Autodesk Fusion 360 part; units mm, degrees
(part 2 of 2)
  line L885 (21.4286, -124.7042) -> (15.7857, -127.9621)
  line L886 (15.7857, -127.9621) -> (15.7857, -134.4779)
  line L887 (21.4286, -137.7358) -> (27.0714, -134.4779)
  line L888 (15.7857, -134.4779) -> (21.4286, -137.7358)
  line L889 (8.6429, -140.3339) -> (8.6429, -146.5)
  line L890 (19.9286, -146.5) -> (19.9286, -140.3339)
  line L891 (14.2857, -137.076) -> (8.6429, -140.3339)
  line L892 (19.9286, -140.3339) -> (14.2857, -137.076)
  line L893 (41.3571, -134.4779) -> (41.3571, -127.9621)
  line L894 (41.3571, -127.9621) -> (35.7143, -124.7042)
  line L895 (35.7143, -124.7042) -> (30.0714, -127.9621)
  line L896 (30.0714, -127.9621) -> (30.0714, -134.4779)
  line L897 (35.7143, -137.7358) -> (41.3571, -134.4779)
  line L898 (30.0714, -134.4779) -> (35.7143, -137.7358)
  line L899 (22.9286, -140.3339) -> (22.9286, -146.5)
  line L900 (34.2143, -146.5) -> (34.2143, -140.3339)
  line L901 (28.5714, -137.076) -> (22.9286, -140.3339)
  line L902 (34.2143, -140.3339) -> (28.5714, -137.076)
  line L903 (55.6428, -134.4779) -> (55.6428, -127.9621)
  line L904 (55.6428, -127.9621) -> (50, -124.7042)
  line L905 (50, -124.7042) -> (44.3571, -127.9621)
  line L906 (44.3571, -127.9621) -> (44.3571, -134.4779)
  line L907 (50, -137.7358) -> (55.6428, -134.4779)
  line L908 (44.3571, -134.4779) -> (50, -137.7358)
  line L909 (37.2143, -140.3339) -> (37.2143, -146.5)
  line L910 (45.9892, -148.2993) -> (48.5, -146.8497)
  line L911 (48.5, -146.8497) -> (48.5, -140.3339)
  line L912 (42.8571, -137.076) -> (37.2143, -140.3339)
  line L913 (48.5, -140.3339) -> (42.8571, -137.076)
  line L914 (69.9286, -134.4779) -> (69.9286, -127.9621)
  line L915 (69.9286, -127.9621) -> (64.2857, -124.7042)
  line L916 (64.2857, -124.7042) -> (58.6429, -127.9621)
  line L917 (58.6429, -127.9621) -> (58.6429, -134.4779)
  line L918 (64.2857, -137.7358) -> (69.9286, -134.4779)
  line L919 (58.6429, -134.4779) -> (64.2857, -137.7358)
  line L920 (51.5, -140.3339) -> (51.5, -146.8497)
  line L921 (51.5, -146.8497) -> (57.1429, -150.1076)
  line L922 (57.1429, -150.1076) -> (62.7857, -146.8497)
  line L923 (62.7857, -146.8497) -> (62.7857, -140.3339)
  line L924 (57.1429, -137.076) -> (51.5, -140.3339)
  line L925 (62.7857, -140.3339) -> (57.1429, -137.076)
  line L926 (84.2142, -134.4779) -> (84.2142, -127.9621)
  line L927 (78.5715, -124.7041) -> (72.9286, -127.9621)
  line L928 (72.9286, -127.9621) -> (72.9286, -134.4779)
  line L929 (78.5714, -137.7358) -> (84.2142, -134.4779)
  line L930 (72.9286, -134.4779) -> (78.5714, -137.7358)
  line L931 (65.7857, -140.3339) -> (65.7857, -146.8497)
  line L932 (65.7857, -146.8497) -> (71.4286, -150.1076)
  line L933 (71.4286, -150.1076) -> (77.0714, -146.8497)
  line L934 (77.0714, -146.8497) -> (77.0714, -140.3339)
  line L935 (71.4286, -137.076) -> (65.7857, -140.3339)
  line L936 (77.0714, -140.3339) -> (71.4286, -137.076)
  line L937 (98.5, -134.4779) -> (98.5, -127.9621)
  line L938 (98.5, -127.9621) -> (92.8572, -124.7042)
  line L939 (87.2142, -127.9621) -> (87.2142, -134.4779)
  line L940 (92.8571, -137.7358) -> (98.5, -134.4779)
  line L941 (87.2142, -134.4779) -> (92.8571, -137.7358)
  line L942 (80.0714, -140.3339) -> (80.0714, -146.8497)
  line L943 (80.0714, -146.8497) -> (85.7143, -150.1076)
  line L944 (85.7143, -150.1076) -> (91.3571, -146.8497)
  line L945 (91.3571, -146.8497) -> (91.3571, -140.3339)
  line L946 (85.7143, -137.076) -> (80.0714, -140.3339)
  line L947 (91.3571, -140.3339) -> (85.7143, -137.076)
  line L948 (94.3571, -140.3339) -> (94.3571, -146.8497)
  line L949 (94.3571, -146.8497) -> (100, -150.1076)
  line L950 (100, -137.076) -> (94.3571, -140.3339)
  line L951 (-87.2143, -154.113) -> (-87.2143, -152.7061)
  line L952 (-87.2143, -152.7061) -> (-92.8572, -149.4482)
  line L953 (-92.8572, -149.4482) -> (-98.143, -152.5)
  line L954 (-72.9286, -159.2219) -> (-72.9286, -152.7061)
  line L955 (-72.9286, -152.7061) -> (-78.5714, -149.4482)
  line L956 (-78.5714, -149.4482) -> (-84.2143, -152.7061)
  line L957 (-84.2143, -152.7061) -> (-84.2143, -159.2219)
  line L958 (-78.5714, -162.4798) -> (-72.9286, -159.2219)
  line L959 (-84.2143, -159.2219) -> (-78.5714, -162.4798)
  line L960 (-80.0714, -170.5) -> (-80.0714, -165.0779)
  line L961 (-80.0714, -165.0779) -> (-85, -162.2324)
  line L962 (-58.6429, -159.2219) -> (-58.6429, -152.7061)
  line L963 (-58.6429, -152.7061) -> (-64.2857, -149.4482)
  line L964 (-64.2857, -149.4482) -> (-69.9286, -152.7061)
  line L965 (-69.9286, -152.7061) -> (-69.9286, -159.2219)
  line L966 (-64.2857, -162.4798) -> (-58.6429, -159.2219)
  line L967 (-69.9286, -159.2219) -> (-64.2857, -162.4798)
  line L968 (-77.0714, -165.0779) -> (-77.0714, -170.5)
  line L969 (-65.7857, -170.5) -> (-65.7857, -165.0779)
  line L970 (-71.4286, -161.82) -> (-77.0714, -165.0779)
  line L971 (-65.7857, -165.0779) -> (-71.4286, -161.82)
  line L972 (-47.6236, -150.8202) -> (-50, -149.4482)
  line L973 (-50, -149.4482) -> (-55.6429, -152.7061)
  line L974 (-55.6429, -152.7061) -> (-55.6429, -159.2219)
  line L975 (-50, -162.4798) -> (-48, -161.3251)
  line L976 (-55.6429, -159.2219) -> (-50, -162.4798)
  line L977 (-62.7857, -165.0779) -> (-62.7857, -170.5)
  line L978 (-51.5, -170.5) -> (-51.5, -165.0779)
  line L979 (-57.1429, -161.82) -> (-62.7857, -165.0779)
  line L980 (-51.5, -165.0779) -> (-57.1429, -161.82)
  line L981 (-48.5, -165.0779) -> (-48.5, -170.5)
  line L982 (55.6428, -159.2219) -> (55.6428, -152.7061)
  line L983 (55.6428, -152.7061) -> (50, -149.4482)
  line L984 (50, -149.4482) -> (47.6236, -150.8202)
  line L985 (50, -162.4798) -> (55.6428, -159.2219)
  line L986 (48, -161.3251) -> (50, -162.4798)
  line L987 (48.5, -170.5) -> (48.5, -165.0779)
  line L988 (69.9286, -159.2219) -> (69.9286, -152.7061)
  line L989 (69.9286, -152.7061) -> (64.2857, -149.4482)
  line L990 (64.2857, -149.4482) -> (58.6429, -152.7061)
  line L991 (58.6429, -152.7061) -> (58.6429, -159.2219)
  line L992 (64.2857, -162.4798) -> (69.9286, -159.2219)
  line L993 (58.6429, -159.2219) -> (64.2857, -162.4798)
  line L994 (51.5, -165.0779) -> (51.5, -170.5)
  line L995 (62.7857, -170.5) -> (62.7857, -165.0779)
  line L996 (57.1429, -161.82) -> (51.5, -165.0779)
  line L997 (62.7857, -165.0779) -> (57.1429, -161.82)
  line L998 (84.2143, -159.2219) -> (84.2143, -152.7061)
  line L999 (84.2143, -152.7061) -> (78.5714, -149.4482)
  line L1000 (78.5714, -149.4482) -> (72.9286, -152.7061)
  line L1001 (72.9286, -152.7061) -> (72.9286, -159.2219)
  line L1002 (78.5714, -162.4798) -> (84.2143, -159.2219)
  line L1003 (72.9286, -159.2219) -> (78.5714, -162.4798)
  line L1004 (65.7857, -165.0779) -> (65.7857, -170.5)
  line L1005 (77.0714, -170.5) -> (77.0714, -165.0779)
  line L1006 (71.4286, -161.82) -> (65.7857, -165.0779)
  line L1007 (77.0714, -165.0779) -> (71.4286, -161.82)
  line L1008 (98.5, -159.2219) -> (98.5, -152.7061)
  line L1009 (98.5, -152.7061) -> (92.8571, -149.4482)
  line L1010 (92.8571, -149.4482) -> (87.2143, -152.7061)
  line L1011 (87.2143, -152.7061) -> (87.2143, -159.2219)
  line L1012 (92.8571, -162.4798) -> (98.5, -159.2219)
  line L1013 (87.2143, -159.2219) -> (92.8571, -162.4798)
  line L1014 (80.0714, -165.0779) -> (80.0714, -170.5)
  line L1015 (91.3571, -170.5) -> (91.3571, -165.0779)
  line L1016 (85.7143, -161.82) -> (80.0714, -165.0779)
  line L1017 (91.3571, -165.0779) -> (85.7143, -161.82)
  line L1018 (94.3571, -165.0779) -> (94.3571, -170.5)
  line L1019 (100, -161.82) -> (94.3571, -165.0779)
  line L1020 (-87.3117, -12.9883) -> (-90.0117, -8.3117)
  line L1021 (-90.0117, -8.3117) -> (-94.6883, -11.0117)
  line L1022 (-94.6883, -11.0117) -> (-91.9883, -15.6883)
  line L1023 (-91.9883, -15.6883) -> (-87.3117, -12.9883)
  line L1024 (14.2857, -87.588) -> (14.2857, -100.6196) construction
  line L1025 (-1.5, -127.9621) -> (-12.7857, -134.4779) construction
  line L1026 (84.2143, -103.2181) -> (72.9286, -109.7339) construction
  line L1027 (62.7857, -47.8737) -> (51.5, -41.3579) construction
  line L1028 (62.7857, -16.6139) -> (51.5, -23.1297) construction
  line L1029 (91.3571, -122.1057) -> (80.0714, -115.5899) construction
  line L1030 (27.0714, -28.9861) -> (15.7857, -35.5019) construction
  line L1031 (-99.7506, -13.5) -> (-92.8571, -17.4799)
  line L1032 (-92.8571, -17.4799) -> (-84.2143, -12.49)
  line L1033 (-84.2143, -12.49) -> (-84.2143, -7.5)
  line L1034 (65.786, -24.8622) -> (65.7862, -14.8818)
  line L1035 (65.7862, -14.8818) -> (57.1431, -9.8914)
  line L1036 (57.1431, -9.8914) -> (48.4997, -14.8814)
  line L1037 (48.4997, -14.8814) -> (48.4995, -24.8617)
  line L1038 (48.4995, -24.8617) -> (57.1426, -29.8521)
  line L1039 (57.1426, -29.8521) -> (65.786, -24.8622)
  line L1040 (30.0714, -37.2339) -> (30.0714, -27.254)
  line L1041 (30.0714, -27.254) -> (21.4285, -22.2641)
  line L1042 (21.4285, -22.2641) -> (12.7857, -27.2541)
  line L1043 (12.7857, -27.2541) -> (12.7857, -37.234)
  line L1044 (12.7857, -37.234) -> (21.4286, -42.2239)
  line L1045 (21.4286, -42.2239) -> (30.0714, -37.2339)
  line L1046 (65.7857, -39.6258) -> (57.1429, -34.6359)
  line L1047 (57.1429, -34.6359) -> (48.5, -39.6258)
  line L1048 (48.5, -39.6258) -> (48.5, -49.6057)
  line L1049 (48.5, -49.6057) -> (57.1429, -54.5957)
  line L1050 (57.1429, -54.5957) -> (65.7857, -49.6057)
  line L1051 (65.7857, -49.6057) -> (65.7857, -39.6258)
  line L1052 (94.3574, -123.8382) -> (94.3576, -113.8578)
  line L1053 (94.3576, -113.8578) -> (87.2143, -109.7334)
  line L1054 (77.0711, -115.5897) -> (77.0709, -123.8377)
  line L1055 (77.0709, -123.8377) -> (85.714, -128.8281)
  line L1056 (85.714, -128.8281) -> (94.3574, -123.8382)
  line L1057 (80.0714, -115.5899) -> (85.7143, -112.332)
  line L1058 (87.2143, -109.7334) -> (87.2143, -101.486)
  line L1059 (87.2143, -101.486) -> (78.5714, -96.4961)
  line L1060 (78.5714, -96.4961) -> (69.9286, -101.486)
  line L1061 (69.9286, -101.486) -> (69.9286, -111.466)
  line L1062 (69.9286, -111.466) -> (77.0711, -115.5897)
  line L1063 (1.5, -136.2099) -> (1.5, -126.23)
  line L1064 (1.5, -126.23) -> (-7.1429, -121.2401)
  line L1065 (-7.1429, -121.2401) -> (-15.7857, -126.2301)
  line L1066 (-15.7857, -126.2301) -> (-15.7857, -136.21)
  line L1067 (-15.7857, -136.21) -> (-7.1429, -141.1999)
  line L1068 (-7.1429, -141.1999) -> (1.5, -136.2099)
  line L1069 (22.9288, -99.0942) -> (22.9291, -89.1138)
  line L1070 (22.9291, -89.1138) -> (14.286, -84.1234)
  line L1071 (14.286, -84.1234) -> (5.6426, -89.1134)
  line L1072 (5.6426, -89.1134) -> (5.6424, -99.0937)
  line L1073 (5.6424, -99.0937) -> (14.2855, -104.0841)
  line L1074 (14.2855, -104.0841) -> (22.9288, -99.0942)
  line L1075 (-30.0714, -53.7301) -> (-41.3571, -60.2459) construction
  line L1076 (-72.9286, -78.4741) -> (-84.2143, -84.9899) construction
  line L1077 (-27.0714, -61.9779) -> (-27.0714, -51.998)
  line L1078 (-27.0714, -51.998) -> (-35.7143, -47.0081)
  line L1079 (-35.7143, -47.0081) -> (-44.3572, -51.9981)
  line L1080 (-44.3572, -51.9981) -> (-44.3571, -61.978)
  line L1081 (-44.3571, -61.978) -> (-35.7143, -66.9679)
  line L1082 (-35.7143, -66.9679) -> (-27.0714, -61.9779)
  line L1083 (-69.9286, -86.7219) -> (-69.9286, -76.742)
  line L1084 (-69.9286, -76.742) -> (-78.5714, -71.7521)
  line L1085 (-78.5714, -71.7521) -> (-87.2143, -76.7421)
  line L1086 (-87.2143, -76.7421) -> (-87.2143, -86.722)
  line L1087 (-87.2143, -86.722) -> (-78.5714, -91.7119)
  line L1088 (-78.5714, -91.7119) -> (-69.9286, -86.7219)
  line L1089 (102.5, -9) -> (99, -9)
  arc A25 (98.5, -8.5) -> (99, -9) centre (99, -8.5) ccw
  line L1090 (98.5, -8.5) -> (98.5, -5)
  line L1091 (96.5, -3) -> (-96.5, -3)
  line L1092 (-98.5, -5) -> (-98.5, -8.5)
  arc A26 (-99, -9) -> (-98.5, -8.5) centre (-99, -8.5) ccw
  line L1093 (-99, -9) -> (-102.5, -9)
  arc A27 (-89.5, -159) -> (-91.5, -157) centre (-91.5, -159) ccw
  arc A28 (-41.5, -151) -> (-43.5, -153) centre (-41.5, -153) ccw
  line L1094 (-41.5, -151) -> (41.5, -151)
  arc A29 (43.5, -153) -> (41.5, -151) centre (41.5, -153) ccw
  line L1095 (43.5, -153) -> (43.5, -173)
  line L1096 (45.5, -175) -> (102.5, -175)
  line L1097 (104.5, -173) -> (104.5, -11)
  line L1098 (84.2143, -109.7339) -> (78.5714, -112.9918)
  line L1099 (48.5, -165.0779) -> (48, -164.7892)
  line L1100 (-48.5, -165.0779) -> (-48, -164.7892)
  line L1101 (-21.4286, -88.2478) -> (-27.0714, -84.9899)
  line L1102 (51.7268, -13.2776) -> (54.4268, -17.9541)
  line L1103 (54.4268, -17.9541) -> (59.1033, -15.2541)
  line L1104 (59.1033, -15.2541) -> (56.4033, -10.5776)
  line L1105 (56.4033, -10.5776) -> (51.7268, -13.2776)
  line L1106 (54.2268, -45.1776) -> (56.9268, -49.8541)
  line L1107 (56.9268, -49.8541) -> (61.6033, -47.1541)
  line L1108 (61.6033, -47.1541) -> (58.9033, -42.4776)
  line L1109 (58.9033, -42.4776) -> (54.2268, -45.1776)
  line L1110 (17.715, -35.1658) -> (23.115, -35.1658)
  line L1111 (23.115, -35.1658) -> (23.115, -29.7658)
  line L1112 (23.115, -29.7658) -> (17.715, -29.7658)
  line L1113 (17.715, -29.7658) -> (17.715, -35.1658)
  line L1114 (17.7151, -91.9658) -> (17.715, -97.3658)
  line L1115 (17.715, -97.3658) -> (23.115, -97.3659)
  line L1116 (23.115, -97.3659) -> (23.1151, -91.9659)
  line L1117 (23.1151, -91.9659) -> (17.7151, -91.9658)
  line L1118 (88.8386, -111.8451) -> (86.1386, -107.1685)
  line L1119 (86.1386, -107.1685) -> (81.4621, -109.8685)
  line L1120 (81.4621, -109.8685) -> (84.1621, -114.5451)
  line L1121 (84.1621, -114.5451) -> (88.8386, -111.8451)
  line L1122 (-9.6883, -133.5117) -> (-6.9883, -138.1883)
  line L1123 (-6.9883, -138.1883) -> (-2.3117, -135.4883)
  line L1124 (-2.3117, -135.4883) -> (-5.0117, -130.8117)
  line L1125 (-5.0117, -130.8117) -> (-9.6883, -133.5117)
  arc A30 (98.5, -5) -> (96.5, -3) centre (96.5, -5) ccw
  arc A31 (104.5, -11) -> (102.5, -9) centre (102.5, -11) ccw
  arc A32 (-96.5, -3) -> (-98.5, -5) centre (-96.5, -5) ccw
  arc A33 (-102.5, -9) -> (-104.5, -11) centre (-102.5, -11) ccw
  arc A34 (43.5, -173) -> (45.5, -175) centre (45.5, -173) ccw
  arc A35 (102.5, -175) -> (104.5, -173) centre (102.5, -173) ccw
  point P0 (-92.8572, -7.5)
  point P1 (-100, -19.8718)
  point P2 (55.415, -14.2658)
  point P3 (57.915, -46.1658)
  point P4 (-6, -134.5)
  point P5 (85.1504, -110.8568)
  point P6 (-91, -12)
  point P7 (85.1504, -110.8568)
  point P8 (-92.8572, -7.5)
  point P9 (57.1429, -19.8718)
  point P10 (21.4286, -32.244)
  point P11 (57.1429, -44.6158)
  point P12 (85.7143, -118.8478)
  point P13 (78.5714, -106.476)
  point P14 (-7.1429, -131.22)
  point P15 (14.2857, -94.1038)
  point P16 (-35.7143, -56.988)
  point P17 (-78.5714, -81.732)
  point P18 (55.415, -14.2658)
  point P19 (57.915, -46.1658)
  point P20 (20.415, -32.4658)
  point P21 (20.415, -94.6658)
  point P22 (85.1504, -110.8568)
  point P23 (-6, -134.5)
  dimension "d9" = 0
  dimension "d44" = 3
  dimension "d57" = 2.7
  dimension "d58" = 30
  dimension "d74" = 2.7
  dimension "d75" = 30
  dimension "d76" = 2.7
  dimension "d77" = 30
  dimension "d78" = 2.7
  dimension "d79" = 2.7
  dimension "d80" = 2.7
  dimension "d81" = 60
  dimension "d82" = 2.7
  dimension "d83" = 30
  dimension "d114" = 2
  dimension "d115" = 2
  dimension "d116" = 2
  dimension "d117" = 2
  dimension "d118" = 2
  dimension "d119" = 2
  constraint coincident L31.start origin
  constraint perpendicular L8 L31
  constraint parallel L29 L31
  constraint coincident L13 P8
  constraint coincident L24 L32.start
  constraint coincident L16 L32.end
  constraint perpendicular L16 L32
  constraint coincident P18 P2
  constraint coincident P19 P3
  constraint coincident P23 P4
  constraint coincident P22 P7
  constraint coincident P6 A13.centre
  constraint coincident P8 P0
  constraint midpoint L1028 P9
  constraint midpoint L1030 P10
  constraint midpoint L1027 P11
  constraint midpoint L1029 P12
  constraint midpoint L1026 P13
  constraint midpoint L1025 P14
  constraint midpoint L1024 P15
  constraint midpoint L1075 P16
  constraint midpoint L1076 P17
  constraint coincident L926.end L1055
  constraint coincident L939.start L1056
  constraint coincident L938.end L1056
  constraint coincident L799.start L1052
  constraint coincident L927.start L1055
  constraint coincident L787.end L1054
  constraint coincident L800.end L1052
  constraint coincident L792.start L1053
  constraint coincident L791.end L1058
  constraint coincident L637.start L1059
  constraint coincident L636.end L1059
  constraint coincident L627.start L1060
  constraint coincident L626.end L1060
  constraint coincident L769.start L1061
  constraint coincident L772.end L1061
  constraint coincident L788.start L1062
  constraint concentric A7 A20
  constraint parallel L7 L12
  constraint parallel L8 L13
  constraint parallel L9 L14
  constraint concentric A10 A21
  constraint parallel L10 L15
  constraint parallel L0 L16
  constraint parallel L1 L17
  constraint concentric A1 A22
  constraint parallel L2 L18
  constraint parallel L3 L19
  constraint parallel L4 L20
  constraint concentric A4 A23
  constraint parallel L5 L21
  constraint concentric A5 A24
  constraint parallel L6 L22
  constraint tangent A24 L22
  constraint tangent A20 L12
  constraint tangent L11 A20
  constraint tangent A21 L15
  constraint tangent L14 A21
  constraint tangent L17 A22
  constraint tangent A22 L18
  constraint tangent L20 A23
  constraint tangent A23 L21
  constraint tangent L21 A24
  constraint coincident L24 L1019.start
  constraint coincident L24 L949.end
  constraint coincident L24 L950.start
  constraint coincident L24 L800.start
  constraint coincident L24 L799.end
  constraint coincident L24 L642.end
  constraint coincident L24 L643.start
  constraint coincident L24 L481.end
  constraint coincident A20 L148.end
  constraint coincident L13 L147.start
  constraint coincident L13 L138.end
  constraint coincident L13 L139.start
  constraint coincident L24 L482.start
  constraint coincident L24 L315.end
  constraint coincident L24 L316.start
  constraint coincident L24 L157.end
  constraint coincident L11 L158.start
  constraint coincident L13 L129.end
  constraint coincident L13 L130.start
  constraint coincident L13 L121.end
  constraint coincident L13 L122.start
  constraint coincident L13 L112.end
  constraint coincident L13 L113.start
  constraint coincident L13 L103.end
  constraint coincident L13 L104.start
  constraint coincident L13 L93.end
  constraint coincident L13 L83.end
  constraint coincident L13 L84.start
  constraint coincident L13 L73.end
  constraint coincident L13 L74.start
  constraint coincident L13 L63.end
  constraint coincident L13 L64.start
  constraint coincident L13 L53.end
  constraint coincident L13 L54.start
  constraint coincident L13 L43.end
  constraint coincident L13 L44.start
  constraint coincident L13 L33.end
  constraint coincident L13 L34.start
  constraint coincident L13 L26.end
  constraint coincident L15 L30.end
  constraint coincident L15 L1031.start
  constraint coincident A22 L951.start
  constraint coincident L17 L953.end
  constraint coincident L18 L961.end
  constraint coincident L19 L960.start
  constraint coincident L19 L968.end
  constraint coincident L19 L969.start
  constraint coincident L19 L977.end
  constraint coincident L19 L978.start
  constraint coincident L19 L981.end
  constraint coincident L20 L975.end
  constraint coincident A23 L972.start
  constraint coincident A23 L853.end
  constraint coincident L21 L854.start
  constraint coincident L21 L862.end
  constraint coincident L21 L863.start
  constraint coincident L21 L872.end
  constraint coincident L21 L873.start
  constraint coincident L21 L881.start
  constraint coincident L21 L880.end
  constraint coincident L21 L900.start
  constraint coincident L21 L899.end
  constraint coincident L21 L890.start
  constraint coincident L21 L889.end
  constraint coincident A24 L910.start
  constraint coincident L21 L909.end
  constraint coincident A24 L984.end
  constraint coincident L22 L986.start
  constraint coincident L23 L987.start
  constraint coincident L22 L1099.end
  constraint coincident L23 L1018.end
  constraint coincident L23 L1015.start
  constraint coincident L23 L1014.end
  constraint coincident L23 L1005.start
  constraint coincident L23 L1004.end
  constraint coincident L23 L995.start
  constraint coincident L23 L994.end
  constraint coincident L20 L1100.end
  constraint coincident L16 L807.start
  constraint coincident L16 L809.end
  constraint coincident L271.end L1045
  constraint coincident L267.start L1045
  constraint coincident L260.end L1044
  constraint coincident L261.start L1044
  constraint coincident L243.end L1043
  constraint coincident L240.start L1043
  constraint coincident L108.end L1042
  constraint coincident L109.start L1042
  constraint coincident L116.end L1041
  constraint coincident L117.start L1041
  constraint coincident L264.end L1040
  constraint coincident L266.start L1040
  constraint coincident L735.end L1074
  constraint coincident L736.start L1074
  constraint coincident L590.start L1069
  constraint coincident L593.end L1069
  constraint coincident L577.start L1070
  constraint coincident L576.end L1070
  constraint coincident L563.start L1071
  constraint coincident L567.end L1071
  constraint coincident L572.start L1072
  constraint coincident L570.end L1072
  constraint coincident L725.start L1073
  constraint coincident L724.end L1073
  constraint coincident L297.start L1051
  constraint coincident L446.end L1050
  constraint coincident L447.start L1050
  constraint coincident L434.end L1049
  constraint coincident L435.start L1049
  constraint coincident L278.end L1048
  constraint coincident L280.start L1048
  constraint coincident L275.end L1047
  constraint coincident L272.start L1047
  constraint coincident L283.end L1046
  constraint coincident L284.start L1046
  constraint coincident L300.end L1051
  constraint coincident L283.start L1039
  constraint coincident L282.end L1039
  constraint coincident L142.start L1034
  constraint coincident L145.end L1034
  constraint coincident L131.start L1035
  constraint coincident L130.end L1035
  constraint coincident L121.start L1036
  constraint coincident L123.end L1036
  constraint coincident L128.start L1037
  constraint coincident L126.end L1037
  constraint coincident L273.start L1038
  constraint coincident L272.end L1038
  constraint coincident L880.start L1068
  constraint coincident L882.end L1068
  constraint coincident L879.start L1063
  constraint coincident L877.end L1063
  constraint coincident L730.start L1064
  constraint coincident L729.end L1064
  constraint coincident L721.start L1065
  constraint coincident L720.end L1065
  constraint coincident L857.start L1066
  constraint coincident L860.end L1066
  constraint coincident L874.start L1067
  constraint coincident L873.end L1067
  constraint coincident L16 L650.start
  constraint coincident L16 L652.end
  constraint coincident L16 L489.start
  constraint coincident L16 L491.end
  constraint coincident L16 L323.start
  constraint coincident L16 L325.end
  constraint coincident L16 L165.start
  constraint coincident L16 L167.end
  constraint coincident L16 L28.start
  constraint coincident P20 A17.centre
  constraint parallel L1043 L1113
  constraint coincident P21 A15.centre
  constraint parallel L1069 L1116
  constraint coincident A21 L27.start
  constraint parallel L11 L1089
  constraint concentric A20 A25
  constraint parallel L12 L1090
  constraint parallel L13 L1091
  constraint parallel L14 L1092
  constraint concentric A21 A26
  constraint parallel L15 L1093
  constraint concentric A22 A27
  constraint concentric A23 A28
  constraint parallel L21 L1094
  constraint concentric A24 A29
  constraint parallel L22 L1095
  constraint parallel L23 L1096
  constraint parallel L24 L1097
  constraint tangent A26 L1093
  constraint tangent A29 L1095
  constraint tangent L1089 A25
  constraint tangent A25 L1090
  constraint tangent L1092 A26
  constraint tangent A28 L1094
  constraint tangent L1094 A29
  constraint tangent L1090 A30
  constraint tangent L1091 A30
  constraint tangent L1097 A31
  constraint tangent L1089 A31
  constraint tangent L1092 A32
  constraint tangent L1091 A32
  constraint tangent L1093 A33
  constraint tangent L1096 A34
  constraint tangent L1095 A34
  constraint tangent L1096 A35
  constraint tangent L1097 A35
  measures "d44" distance of L27 L30
  measures "d57" distance of P6 L1023
  measures "d58" angle of L13 L1021
  measures "d74" distance of P18 L1105
  measures "d75" angle of L1091 L1105
  measures "d76" distance of P19 L1109
  measures "d77" angle of L24 L1106
  measures "d78" distance of P20 L1113
  measures "d79" distance of P21 L1117
  measures "d80" distance of P22 L1121
  measures "d81" angle of L24 L1121
  measures "d82" distance of P23 L1125
  measures "d83" angle of L1094 L1123
  measures "d114" radius of A30
  measures "d115" radius of A31
  measures "d116" radius of A32
  measures "d117" radius of A33
  measures "d118" radius of A34
  measures "d119" radius of A35
extrude "Extrude4" add sketch "Sketch1" along normal blind 1.4 contours L0 A0 L1 A1 L2 A2 L3 A3 L4 A4 L5 A5 L6 A6 A7 L7 A8 L8 A9 L9 A10 L10 A11 L1089 A25 L1090 L1091 L1092 A26 L1093 A27 A28 L1094 A29 L1095 L1096 L1097 A30 A31 A32 A33 A34 A35 | L13 L14 A21 L25 L26 L1020 L1021 | L13 A21 L15 L25 L26 L27 L30 L34 L41 L1020 L1022 L1023 L1031 L1032 L1033 | A21 L27 L1022 | A21 L1021 L1022 | L11 A20 L13 L16 L17 A22 L18 L19 L20 A23 L21 A24 L22 L23 L24 L28 L29 L33 L35 L36 L37 L38 L39 L40 L42 L43 L44 L45 L46 L53 L54 L55 L56 L63 L64 L65 L66 L73 L74 L75 L76 L83 L84 L85 L86 L93 L94 L95 L96 L103 L104 L105 L106 L112 L113 L114 L115 L122 L123 L124 L125 L126 L127 L128 L129 L131 L138 L139 L140 L141 L142 L143 L144 L145 L146 L147 L148 L149 L156 L157 L158 L165 L166 L167 L273 L274 L275 L276 L277 L278 L279 L280 L281 L282 L284 L297 L298 L299 L300 L301 L314 L315 L316 L323 L324 L325 L434 L435 L436 L437 L438 L445 L446 L447 L448 L449 L480 L481 L482 L489 L490 L491 L625 L626 L627 L628 L629 L636 L637 L638 L639 L640 L641 L642 L643 L650 L651 L652 L719 L720 L721 L722 L723 L729 L730 L731 L732 L733 L769 L770 L771 L772 L773 L785 L786 L787 L788 L789 L790 L791 L792 L799 L800 L807 L808 L809 L852 L853 L854 L855 L856 L857 L858 L859 L860 L861 L862 L863 L864 L865 L872 L874 L875 L876 L877 L878 L879 L881 L882 L889 L890 L891 L892 L899 L900 L901 L902 L909 L910 L911 L912 L913 L926 L927 L928 L929 L930 L937 L938 L939 L940 L941 L948 L949 L950 L951 L952 L953 L960 L961 L968 L969 L970 L971 L972 L973 L974 L975 L976 L977 L978 L979 L980 L981 L982 L983 L984 L985 L986 L987 L994 L995 L996 L997 L1004 L1005 L1006 L1007 L1014 L1015 L1016 L1017 L1018 L1019 L1031 L1032 L1033 L1034 L1035 L1036 L1037 L1038 L1039 L1046 L1047 L1048 L1049 L1050 L1051 L1052 L1053 L1054 L1055 L1056 L1058 L1059 L1060 L1061 L1062 L1063 L1064 L1065 L1066 L1067 L1068 L1099 L1100 | L13 L121 L130 L1035 L1036 | L1034 L1035 L1036 L1037 L1038 L1039 | L272 L283 L1038 L1039 L1046 L1047 | L19 L20 L981 L1100 | L1046 L1047 L1048 L1049 L1050 L1051 | L21 L873 L880 L1067 L1068 | L780 L781 L782 L783 L784 L793 L794 L795 L796 L797 L798 L1052 L1053 L1054 L1055 L1056 L1057 L1058 L1059 L1060 L1061 L1062 L1098 L1118 L1119 L1120 L1121 | L1063 L1064 L1065 L1066 L1067 L1068 | L793 L794 L795 L796 L797 L798 L1057 L1120 L1121 | L780 L781 L782 L783 L784 L1098 L1119 L1120 | L578 L579 L580 L581 L582 L583 L1114 L1115 L1117 | L578 L579 L580 L581 L582 L583 L1069 L1070 L1071 L1072 L1073 L1074 L1115 L1117 | L590 L1069 L1115 | L132 L133 L134 L135 L136 L137 L1102 L1103 L1104 | L1040 L1041 L1042 L1043 L1044 L1045 | L212 L223 L350 L373 L377 L384 L1077 L1078 L1079 L1080 L1081 L1082 | L251 L252 L253 L254 L255 L256 | L285 L286 L287 L288 L289 L290 | L334 L345 L483 L503 L507 L514 L1083 L1084 L1085 L1086 L1087 L1088 | L362 L363 L364 L365 L366 L367 | L492 L493 L494 L495 L496 L497 | L866 L867 L868 L869 L870 L871 L1122 L1124 L1125
extrude "Extrude5" add sketch "Sketch1" against normal blind 1 contours L13 L14 A21 L25 L26 L1020 L1021 | L13 A21 L15 L25 L26 L27 L30 L34 L41 L1020 L1022 L1023 L1031 L1032 L1033 | A21 L27 L1022 | L1034 L1035 L1036 L1037 L1038 L1039 | L1046 L1047 L1048 L1049 L1050 L1051 | L780 L781 L782 L783 L784 L793 L794 L795 L796 L797 L798 L1052 L1053 L1054 L1055 L1056 L1057 L1058 L1059 L1060 L1061 L1062 L1098 L1118 L1119 L1120 L1121 | L1063 L1064 L1065 L1066 L1067 L1068 | L793 L794 L795 L796 L797 L798 L1057 L1120 L1121 | L780 L781 L782 L783 L784 L1098 L1119 L1120 | L578 L579 L580 L581 L582 L583 L1114 L1115 L1117 | L578 L579 L580 L581 L582 L583 L1069 L1070 L1071 L1072 L1073 L1074 L1115 L1117 | L132 L133 L134 L135 L136 L137 L1102 L1103 L1104 | L1040 L1041 L1042 L1043 L1044 L1045 | L212 L223 L350 L373 L377 L384 L1077 L1078 L1079 L1080 L1081 L1082 | L251 L252 L253 L254 L255 L256 | L285 L286 L287 L288 L289 L290 | L334 L345 L483 L503 L507 L514 L1083 L1084 L1085 L1086 L1087 L1088 | L362 L363 L364 L365 L366 L367 | L492 L493 L494 L495 L496 L497 | L866 L867 L868 L869 L870 L871 L1122 L1124 L1125
extrude "Extrude6" add sketch "Sketch1" against normal blind 2 from surface at -1 contours A13 A19 L25 L27 L1020 L1022 L1023 | A13 A19 A21 L25 L27 L1020 L1021 L1022 | L13 L14 A21 L25 L26 L1020 L1021 | L13 A21 L15 L25 L26 L27 L30 L34 L41 L1020 L1022 L1023 L1031 L1032 L1033 | A21 L27 L1022 | L1034 L1035 L1036 L1037 L1038 L1039 | L1046 L1047 L1048 L1049 L1050 L1051 | L780 L781 L782 L783 L784 L793 L794 L795 L796 L797 L798 L1052 L1053 L1054 L1055 L1056 L1057 L1058 L1059 L1060 L1061 L1062 L1098 L1118 L1119 L1120 L1121 | L1063 L1064 L1065 L1066 L1067 L1068 | A14 L780 L798 L1053 L1058 L1118 L1119 L1121 | A14 L797 L798 L1057 L1120 L1121 | L793 L794 L795 L796 L797 L798 L1057 L1120 L1121 | L780 L781 L782 L783 L784 L1098 L1119 L1120 | A14 L780 L1098 L1119 L1120 | A14 L797 L1057 L1098 L1120 | A15 L580 L581 L1069 L1115 L1117 | A15 L580 L581 L1114 L1115 L1117 | L578 L579 L580 L581 L582 L583 L1114 L1115 L1117 | L578 L579 L580 L581 L582 L583 L1069 L1070 L1071 L1072 L1073 L1074 L1115 L1117 | A18 L136 L137 L1102 L1103 L1104 | A18 L136 L137 L1102 L1104 L1105 | L132 L133 L134 L135 L136 L137 L1102 L1103 L1104 | L1040 L1041 L1042 L1043 L1044 L1045 | L212 L223 L350 L373 L377 L384 L1077 L1078 L1079 L1080 L1081 L1082 | L251 L252 L253 L254 L255 L256 | L285 L286 L287 L288 L289 L290 | L334 L345 L483 L503 L507 L514 L1083 L1084 L1085 L1086 L1087 L1088 | L362 L363 L364 L365 L366 L367 | L492 L493 L494 L495 L496 L497 | L866 L867 L868 L869 L870 L871 L1122 L1124 L1125 | L870 L871 L1122 L1123 L1124 | L870 L871 L1122 L1124 L1125 | L1106 L1107 L1108 L1109 | L1110 L1111 L1112 L1113
extrude "Extrude7" cut 1 faces at (5.4294, 137.2883, 85.8) along direction (-0.5, 0.866025, 0) blind 5
extrude "Extrude8" cut 1 faces at (88.8706, 13.8883, 86.6) along direction (-0.5, 0.866025, 0) blind 3
extrude "Extrude9" cut 1 faces at (-17.715, 31.5658, 85.8) along direction (1, 0.000001, 0) blind 7
extrude "Extrude10" cut 1 faces at (-60.0445, 48.0541, 86.6) along direction (-0.5, 0.866025, 0) blind 5.5
extrude "Extrude11" cut 1 faces at (-54.8445, 11.4776, 85.8) along direction (0.5, -0.866025, 0) blind 5.4
extrude "Extrude12" cut 2 faces at (-86.8557, 108.4106, 85.8) (-88.4998, 111.2581, 85.8) along direction (-0.866025, -0.5, 0) blind 3
sketch "Sketch4" plane through (0, 0, 86) normal (0, 0, 1) x (-1, 0, 0)
  line L0 (-96.5, -3) -> (96.5, -3)
  line L1 (104.5, -11) -> (104.5, -173)
  line L2 (-104.5, -155) -> (-104.5, -11)
  line L3 (96.5, -3) -> (-96.5, -3)
  line L4 (104.5, -173) -> (104.5, -11)
  line L5 (-104.5, -9) -> (-104.5, -157)
  line L6 (-89.5, -175) -> (-43.5, -175)
  line L7 (43.5, -173) -> (43.5, -153)
  line L8 (41.5, -151) -> (-41.5, -151)
  line L9 (-43.5, -153) -> (-43.5, -173)
  line L10 (-41.5, -151) -> (41.5, -151)
  line L11 (43.5, -153) -> (43.5, -173)
  line L12 (-102.5, -157) -> (-91.5, -157)
  line L13 (-89.5, -159) -> (-89.5, -173)
  line L14 (-98.5, -5) -> (-98.5, -8.5)
  line L15 (-99, -9) -> (-102.5, -9)
  line L16 (102.5, -9) -> (99, -9)
  line L17 (98.5, -8.5) -> (98.5, -5)
  line L18 (102.5, -175) -> (45.5, -175)
  line L19 (-45.5, -175) -> (-87.5, -175)
  arc A0 (98.5, -5) -> (96.5, -3) centre (96.5, -5) ccw
  arc A1 (43.5, -153) -> (41.5, -151) centre (41.5, -153) ccw
  arc A2 (-41.5, -151) -> (-43.5, -153) centre (-41.5, -153) ccw
  arc A3 (-45.5, -175) -> (-43.5, -173) centre (-45.5, -173) ccw
  arc A4 (-89.5, -173) -> (-87.5, -175) centre (-87.5, -173) ccw
  arc A5 (-89.5, -159) -> (-91.5, -157) centre (-91.5, -159) ccw
  arc A6 (-104.5, -155) -> (-102.5, -157) centre (-102.5, -155) ccw
  arc A7 (-102.5, -9) -> (-104.5, -11) centre (-102.5, -11) ccw
  arc A8 (-99, -9) -> (-98.5, -8.5) centre (-99, -8.5) ccw
  arc A9 (-96.5, -3) -> (-98.5, -5) centre (-96.5, -5) ccw
  arc A10 (98.5, -8.5) -> (99, -9) centre (99, -8.5) ccw
  arc A11 (104.5, -11) -> (102.5, -9) centre (102.5, -11) ccw
  arc A12 (102.5, -175) -> (104.5, -173) centre (102.5, -173) ccw
  arc A13 (43.5, -173) -> (45.5, -175) centre (45.5, -173) ccw
  dimension "d103" = 2
  dimension "d104" = 2
  dimension "d105" = 2
  dimension "d106" = 2
  dimension "d107" = 2
  dimension "d108" = 0.5
  dimension "d109" = 2
  dimension "d110" = 0.5
  dimension "d111" = 2
  dimension "d112" = 2
  dimension "d113" = 2
  constraint horizontal L0
  constraint vertical L1
  constraint horizontal L18
  constraint vertical L2
  constraint collinear L0 L3
  constraint collinear L1 L4
  constraint collinear L2 L5
  constraint collinear L6 L18
  constraint vertical L7
  constraint horizontal L8
  constraint vertical L9
  constraint collinear L8 L10
  constraint collinear L7 L11
  constraint horizontal L12
  constraint vertical L13
  constraint vertical L14
  constraint horizontal L15
  constraint horizontal L16
  constraint vertical L17
  constraint collinear L18 L19
  constraint tangent L0 A0
  constraint tangent L17 A0
  constraint tangent L8 A1
  constraint tangent L7 A1
  constraint equal A0 A1
  constraint tangent L8 A2
  constraint tangent L9 A2
  constraint equal A0 A2
  constraint tangent L19 A3
  constraint tangent L9 A3
  constraint tangent L13 A4
  constraint tangent L19 A4
  constraint tangent L12 A5
  constraint tangent L13 A5
  constraint tangent L2 A6
  constraint tangent L12 A6
  constraint tangent L15 A7
  constraint tangent L2 A7
  constraint equal A6 A7
  constraint tangent L15 A8
  constraint tangent L14 A8
  constraint tangent L0 A9
  constraint tangent L14 A9
  constraint tangent L17 A10
  constraint tangent L16 A10
  constraint tangent L16 A11
  constraint tangent L1 A11
  constraint tangent L18 A12
  constraint tangent L1 A12
  constraint tangent L7 A13
  constraint tangent L18 A13
  measures "d103" radius of A0
  measures "d104" radius of A3
  measures "d105" radius of A4
  measures "d106" radius of A5
  measures "d107" radius of A6
  measures "d108" radius of A8
  measures "d109" radius of A9
  measures "d110" radius of A10
  measures "d111" radius of A11
  measures "d112" radius of A12
  measures "d113" radius of A13
extrude "Extrude13" add sketch "Sketch4" along normal blind 1.6 from surface at 1.4
sketch "Sketch5" plane through (0, 0, 83) normal (0, 0, -1) x (1, 0, 0)
  circle A0 centre (-20.415, -94.6658) radius 1.7
  line L0 (-22.9288, -99.0942) -> (-14.2855, -104.0841)
  line L1 (-14.2855, -104.0841) -> (-5.6424, -99.0937)
  line L2 (-5.6424, -99.0937) -> (-5.6426, -89.1134)
  line L3 (-5.6426, -89.1134) -> (-14.286, -84.1234)
  line L4 (-14.286, -84.1234) -> (-22.9291, -89.1138)
  line L5 (-22.9291, -89.1138) -> (-22.9288, -99.0942)
  circle A1 centre (-55.415, -14.2658) radius 2.5
  circle A2 centre (-57.915, -46.1658) radius 2.5
  circle A3 centre (-20.415, -32.4658) radius 2.5
  circle A4 centre (-20.415, -94.6658) radius 2.5
  circle A5 centre (-85.1504, -110.8568) radius 2.5
  circle A6 centre (-85.1504, -110.8568) radius 1.7
  circle A7 centre (6, -134.5) radius 1.75
  circle A8 centre (-57.915, -46.1658) radius 1.7
  circle A9 centre (-55.415, -14.2658) radius 1.7
  circle A10 centre (-20.415, -32.4658) radius 1.7
  circle A11 centre (91, -12) radius 1.75
  dimension "d123" = 5
  constraint concentric A0 A4
  constraint concentric A5 A6
  constraint concentric A2 A8
  constraint concentric A1 A9
  constraint concentric A3 A10
  constraint equal A1 A3
  constraint equal A2 A3
  constraint equal A2 A5
  constraint equal A4 A5
  measures "d123" diameter of A4
extrude "Extrude14" add sketch "Sketch5" along normal blind 4 contours A1 | A2 | A3 | A4 | A5
extrude "Extrude15" add 4 faces at (75.6904, 80.646, 83) (32.8333, 55.902, 83) (85.9506, 10.4102, 83) (9.856, 126.7804, 83) along direction (0, 0, -1) blind 2
